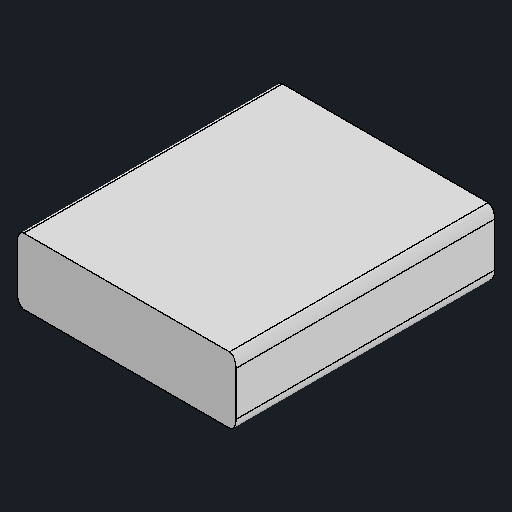
# Autodesk Inventor part: DAC
Saved by Autodesk Inventor 2026.2 (Build 302298000, 298)
## iProperties
Created: 2026-06-15
Part Number: DAC
Material: Generic
Document SubType Name: Modeling
Designer: JoshuaEah
Density: 1 g/cm^3
Appearance: Default
Author: JoshuaEah
Autodesk Inventor part; units mm, degrees
ref_plane "YZ Plane" through (0, 0, 0) normal (1, 0, 0) x (0, 1, 0)
ref_plane "XZ Plane" through (0, 0, 0) normal (0, 1, 0) x (-1, 0, 0)
ref_plane "XY Plane" through (0, 0, 0) normal (0, 0, 1) x (1, 0, 0)
sketch "Sketch1" plane through (0, 0, 0) normal (0, 0, 1) x (1, 0, 0)
  line L0 (0, 0) -> (100, 0)
  line L1 (100, 0) -> (100, 30.2)
  line L2 (100, 30.2) -> (0, 30.2)
  line L3 (0, 30.2) -> (0, 0)
  ellipse E0 centre (3, 25.2) end of major axis (0, 25.2) minor radius 5 (3, 30.2) -> (0, 25.2) ccw
  line L4 (50, 30.2) -> (50, 0) construction
  line L5 (0, 15.1) -> (100, 15.1) construction
  ellipse E1 centre (97, 25.2) end of major axis (100, 25.2) minor radius 5 (100, 25.2) -> (97, 30.2) ccw
  ellipse E2 centre (3, 5) end of major axis (0, 5) minor radius 5 (0, 5) -> (3, 0) ccw
  ellipse E3 centre (97, 5) end of major axis (100, 5) minor radius 5 (97, 0) -> (100, 5) ccw
  point P0 (0, 5)
  point P1 (3, 0)
  point P2 (97, 0)
  point P3 (100, 5)
  point P4 (100, 25.2)
  dimension "d0" = 100
  dimension "d1" = 30.2
  dimension "d6" = 3
  dimension "d7" = 5
  constraints: 12 end point, 9 symmetric about line, 4 horizontal, 4 midpoint, 2 parallel, 2 point on line, 2 vertical, 1 coincident, 1 perpendicular, 16 other
  measures "d0" distance of L2.end L1.end
  measures "d1" distance of L1.end L0.end
  measures "d6" distance from line of L3 point (3, 25.2)
  measures "d7" distance from line of L2 point (3, 25.2)
extrude "Extrusion1" add sketch "Sketch1" against normal blind 118.2 contours E2 L3 E0 L2 E1 L1 E3 L0
body "Solid1"
